Autodesk Inventor part; units mm, degrees
(part 4 of 13)
  line L1457 (42.6451, -0.0639) -> (42.8452, 0.1364) construction
  line L1458 (42.8452, 0.1364) -> (42.8452, 0.3832) construction
  spline S448 degree 3 poles (35.1829, 2.9373) (35.1829, 3.1841) (34.9826, 3.3841) (34.7358, 3.3841) knots 0 0 0 0 1 1 1 1
  line L1459 (35.1829, 2.9373) -> (35.1829, 3.1841) construction
  line L1460 (35.1829, 3.1841) -> (34.9826, 3.3841) construction
  line L1461 (34.9826, 3.3841) -> (34.7358, 3.3841) construction
  spline S449 degree 3 poles (34.7358, 3.3841) (34.4891, 3.3841) (34.289, 3.1841) (34.289, 2.9373) knots 0 0 0 0 1 1 1 1
  line L1462 (34.7358, 3.3841) -> (34.4891, 3.3841) construction
  line L1463 (34.4891, 3.3841) -> (34.289, 3.1841) construction
  line L1464 (34.289, 3.1841) -> (34.289, 2.9373) construction
  spline S450 degree 3 poles (34.289, 2.9373) (34.289, 2.6905) (34.4891, 2.4902) (34.7358, 2.4902) knots 0 0 0 0 1 1 1 1
  line L1465 (34.289, 2.9373) -> (34.289, 2.6905) construction
  line L1466 (34.289, 2.6905) -> (34.4891, 2.4902) construction
  line L1467 (34.4891, 2.4902) -> (34.7358, 2.4902) construction
  spline S451 degree 3 poles (34.7358, 2.4902) (34.9826, 2.4902) (35.1829, 2.6905) (35.1829, 2.9373) knots 0 0 0 0 1 1 1 1
  line L1468 (34.7358, 2.4902) -> (34.9826, 2.4902) construction
  line L1469 (34.9826, 2.4902) -> (35.1829, 2.6905) construction
  line L1470 (35.1829, 2.6905) -> (35.1829, 2.9373) construction
  spline S452 degree 3 poles (35.1829, 5.4914) (35.1829, 5.7382) (34.9826, 5.9382) (34.7358, 5.9382) knots 0 0 0 0 1 1 1 1
  line L1471 (35.1829, 5.4914) -> (35.1829, 5.7382) construction
  line L1472 (35.1829, 5.7382) -> (34.9826, 5.9382) construction
  line L1473 (34.9826, 5.9382) -> (34.7358, 5.9382) construction
  spline S453 degree 3 poles (34.7358, 5.9382) (34.4891, 5.9382) (34.289, 5.7382) (34.289, 5.4914) knots 0 0 0 0 1 1 1 1
  line L1474 (34.7358, 5.9382) -> (34.4891, 5.9382) construction
  line L1475 (34.4891, 5.9382) -> (34.289, 5.7382) construction
  line L1476 (34.289, 5.7382) -> (34.289, 5.4914) construction
  spline S454 degree 3 poles (34.289, 5.4914) (34.289, 5.2446) (34.4891, 5.0443) (34.7358, 5.0443) knots 0 0 0 0 1 1 1 1
  line L1477 (34.289, 5.4914) -> (34.289, 5.2446) construction
  line L1478 (34.289, 5.2446) -> (34.4891, 5.0443) construction
  line L1479 (34.4891, 5.0443) -> (34.7358, 5.0443) construction
  spline S455 degree 3 poles (34.7358, 5.0443) (34.9826, 5.0443) (35.1829, 5.2446) (35.1829, 5.4914) knots 0 0 0 0 1 1 1 1
  line L1480 (34.7358, 5.0443) -> (34.9826, 5.0443) construction
  line L1481 (34.9826, 5.0443) -> (35.1829, 5.2446) construction
  line L1482 (35.1829, 5.2446) -> (35.1829, 5.4914) construction
  spline S456 degree 3 poles (37.737, 5.4914) (37.737, 5.7382) (37.5369, 5.9382) (37.29, 5.9382) knots 0 0 0 0 1 1 1 1
  line L1483 (37.737, 5.4914) -> (37.737, 5.7382) construction
  line L1484 (37.737, 5.7382) -> (37.5369, 5.9382) construction
  line L1485 (37.5369, 5.9382) -> (37.29, 5.9382) construction
  spline S457 degree 3 poles (37.29, 5.9382) (37.0431, 5.9382) (36.843, 5.7382) (36.843, 5.4914) knots 0 0 0 0 1 1 1 1
  line L1486 (37.29, 5.9382) -> (37.0431, 5.9382) construction
  line L1487 (37.0431, 5.9382) -> (36.843, 5.7382) construction
  line L1488 (36.843, 5.7382) -> (36.843, 5.4914) construction
  spline S458 degree 3 poles (36.843, 5.4914) (36.843, 5.2446) (37.0431, 5.0443) (37.29, 5.0443) knots 0 0 0 0 1 1 1 1
  line L1489 (36.843, 5.4914) -> (36.843, 5.2446) construction
  line L1490 (36.843, 5.2446) -> (37.0431, 5.0443) construction
  line L1491 (37.0431, 5.0443) -> (37.29, 5.0443) construction
  spline S459 degree 3 poles (37.29, 5.0443) (37.5369, 5.0443) (37.737, 5.2446) (37.737, 5.4914) knots 0 0 0 0 1 1 1 1
  line L1492 (37.29, 5.0443) -> (37.5369, 5.0443) construction
  line L1493 (37.5369, 5.0443) -> (37.737, 5.2446) construction
  line L1494 (37.737, 5.2446) -> (37.737, 5.4914) construction
  spline S460 degree 3 poles (37.737, 0.3832) (37.737, 0.6299) (37.5369, 0.83) (37.29, 0.83) knots 0 0 0 0 1 1 1 1
  line L1495 (37.737, 0.3832) -> (37.737, 0.6299) construction
  line L1496 (37.737, 0.6299) -> (37.5369, 0.83) construction
  line L1497 (37.5369, 0.83) -> (37.29, 0.83) construction
  spline S461 degree 3 poles (37.29, 0.83) (37.0431, 0.83) (36.843, 0.6299) (36.843, 0.3832) knots 0 0 0 0 1 1 1 1
  line L1498 (37.29, 0.83) -> (37.0431, 0.83) construction
  line L1499 (37.0431, 0.83) -> (36.843, 0.6299) construction
  line L1500 (36.843, 0.6299) -> (36.843, 0.3832) construction
  spline S462 degree 3 poles (36.843, 0.3832) (36.843, 0.1364) (37.0431, -0.0639) (37.29, -0.0639) knots 0 0 0 0 1 1 1 1
  line L1501 (36.843, 0.3832) -> (36.843, 0.1364) construction
  line L1502 (36.843, 0.1364) -> (37.0431, -0.0639) construction
  line L1503 (37.0431, -0.0639) -> (37.29, -0.0639) construction
  spline S463 degree 3 poles (37.29, -0.0639) (37.5369, -0.0639) (37.737, 0.1364) (37.737, 0.3832) knots 0 0 0 0 1 1 1 1
  line L1504 (37.29, -0.0639) -> (37.5369, -0.0639) construction
  line L1505 (37.5369, -0.0639) -> (37.737, 0.1364) construction
  line L1506 (37.737, 0.1364) -> (37.737, 0.3832) construction
  spline S464 degree 3 poles (40.2911, 0.3832) (40.2911, 0.6299) (40.091, 0.83) (39.8441, 0.83) knots 0 0 0 0 1 1 1 1
  line L1507 (40.2911, 0.3832) -> (40.2911, 0.6299) construction
  line L1508 (40.2911, 0.6299) -> (40.091, 0.83) construction
  line L1509 (40.091, 0.83) -> (39.8441, 0.83) construction
  spline S465 degree 3 poles (39.8441, 0.83) (39.5972, 0.83) (39.3971, 0.6299) (39.3971, 0.3832) knots 0 0 0 0 1 1 1 1
  line L1510 (39.8441, 0.83) -> (39.5972, 0.83) construction
  line L1511 (39.5972, 0.83) -> (39.3971, 0.6299) construction
  line L1512 (39.3971, 0.6299) -> (39.3971, 0.3832) construction
  spline S466 degree 3 poles (39.3971, 0.3832) (39.3971, 0.1364) (39.5972, -0.0639) (39.8441, -0.0639) knots 0 0 0 0 1 1 1 1
  line L1513 (39.3971, 0.3832) -> (39.3971, 0.1364) construction
  line L1514 (39.3971, 0.1364) -> (39.5972, -0.0639) construction
  line L1515 (39.5972, -0.0639) -> (39.8441, -0.0639) construction
  spline S467 degree 3 poles (39.8441, -0.0639) (40.091, -0.0639) (40.2911, 0.1364) (40.2911, 0.3832) knots 0 0 0 0 1 1 1 1
  line L1516 (39.8441, -0.0639) -> (40.091, -0.0639) construction
  line L1517 (40.091, -0.0639) -> (40.2911, 0.1364) construction
  line L1518 (40.2911, 0.1364) -> (40.2911, 0.3832) construction
  spline S468 degree 3 poles (37.737, 2.9373) (37.737, 3.1841) (37.5369, 3.3841) (37.29, 3.3841) knots 0 0 0 0 1 1 1 1
  line L1519 (37.737, 2.9373) -> (37.737, 3.1841) construction
  line L1520 (37.737, 3.1841) -> (37.5369, 3.3841) construction
  line L1521 (37.5369, 3.3841) -> (37.29, 3.3841) construction
  spline S469 degree 3 poles (37.29, 3.3841) (37.0431, 3.3841) (36.843, 3.1841) (36.843, 2.9373) knots 0 0 0 0 1 1 1 1
  line L1522 (37.29, 3.3841) -> (37.0431, 3.3841) construction
  line L1523 (37.0431, 3.3841) -> (36.843, 3.1841) construction
  line L1524 (36.843, 3.1841) -> (36.843, 2.9373) construction
  spline S470 degree 3 poles (36.843, 2.9373) (36.843, 2.6905) (37.0431, 2.4902) (37.29, 2.4902) knots 0 0 0 0 1 1 1 1
  line L1525 (36.843, 2.9373) -> (36.843, 2.6905) construction
  line L1526 (36.843, 2.6905) -> (37.0431, 2.4902) construction
  line L1527 (37.0431, 2.4902) -> (37.29, 2.4902) construction
  spline S471 degree 3 poles (37.29, 2.4902) (37.5369, 2.4902) (37.737, 2.6905) (37.737, 2.9373) knots 0 0 0 0 1 1 1 1
  line L1528 (37.29, 2.4902) -> (37.5369, 2.4902) construction
  line L1529 (37.5369, 2.4902) -> (37.737, 2.6905) construction
  line L1530 (37.737, 2.6905) -> (37.737, 2.9373) construction
  spline S472 degree 3 poles (35.1829, 8.0455) (35.1829, 8.2923) (34.9826, 8.4923) (34.7358, 8.4923) knots 0 0 0 0 1 1 1 1
  line L1531 (35.1829, 8.0455) -> (35.1829, 8.2923) construction
  line L1532 (35.1829, 8.2923) -> (34.9826, 8.4923) construction
  line L1533 (34.9826, 8.4923) -> (34.7358, 8.4923) construction
  spline S473 degree 3 poles (34.7358, 8.4923) (34.4891, 8.4923) (34.289, 8.2923) (34.289, 8.0455) knots 0 0 0 0 1 1 1 1
  line L1534 (34.7358, 8.4923) -> (34.4891, 8.4923) construction
  line L1535 (34.4891, 8.4923) -> (34.289, 8.2923) construction
  line L1536 (34.289, 8.2923) -> (34.289, 8.0455) construction
  spline S474 degree 3 poles (34.289, 8.0455) (34.289, 7.7987) (34.4891, 7.5984) (34.7358, 7.5984) knots 0 0 0 0 1 1 1 1
  line L1537 (34.289, 8.0455) -> (34.289, 7.7987) construction
  line L1538 (34.289, 7.7987) -> (34.4891, 7.5984) construction
  line L1539 (34.4891, 7.5984) -> (34.7358, 7.5984) construction
  spline S475 degree 3 poles (34.7358, 7.5984) (34.9826, 7.5984) (35.1829, 7.7987) (35.1829, 8.0455) knots 0 0 0 0 1 1 1 1
  line L1540 (34.7358, 7.5984) -> (34.9826, 7.5984) construction
  line L1541 (34.9826, 7.5984) -> (35.1829, 7.7987) construction
  line L1542 (35.1829, 7.7987) -> (35.1829, 8.0455) construction
  spline S476 degree 3 poles (37.737, 8.0455) (37.737, 8.2923) (37.5369, 8.4923) (37.29, 8.4923) knots 0 0 0 0 1 1 1 1
  line L1543 (37.737, 8.0455) -> (37.737, 8.2923) construction
  line L1544 (37.737, 8.2923) -> (37.5369, 8.4923) construction
  line L1545 (37.5369, 8.4923) -> (37.29, 8.4923) construction
  spline S477 degree 3 poles (37.29, 8.4923) (37.0431, 8.4923) (36.843, 8.2923) (36.843, 8.0455) knots 0 0 0 0 1 1 1 1
  line L1546 (37.29, 8.4923) -> (37.0431, 8.4923) construction
  line L1547 (37.0431, 8.4923) -> (36.843, 8.2923) construction
  line L1548 (36.843, 8.2923) -> (36.843, 8.0455) construction
  spline S478 degree 3 poles (36.843, 8.0455) (36.843, 7.7987) (37.0431, 7.5984) (37.29, 7.5984) knots 0 0 0 0 1 1 1 1
  line L1549 (36.843, 8.0455) -> (36.843, 7.7987) construction
  line L1550 (36.843, 7.7987) -> (37.0431, 7.5984) construction
  line L1551 (37.0431, 7.5984) -> (37.29, 7.5984) construction
  spline S479 degree 3 poles (37.29, 7.5984) (37.5369, 7.5984) (37.737, 7.7987) (37.737, 8.0455) knots 0 0 0 0 1 1 1 1
  line L1552 (37.29, 7.5984) -> (37.5369, 7.5984) construction
  line L1553 (37.5369, 7.5984) -> (37.737, 7.7987) construction
  line L1554 (37.737, 7.7987) -> (37.737, 8.0455) construction
  spline S480 degree 3 poles (35.1829, 10.5996) (35.1829, 10.8464) (34.9826, 11.0465) (34.7358, 11.0465) knots 0 0 0 0 1 1 1 1
  line L1555 (35.1829, 10.5996) -> (35.1829, 10.8464) construction
  line L1556 (35.1829, 10.8464) -> (34.9826, 11.0465) construction
  line L1557 (34.9826, 11.0465) -> (34.7358, 11.0465) construction
  spline S481 degree 3 poles (34.7358, 11.0465) (34.4891, 11.0465) (34.289, 10.8464) (34.289, 10.5996) knots 0 0 0 0 1 1 1 1
  line L1558 (34.7358, 11.0465) -> (34.4891, 11.0465) construction
  line L1559 (34.4891, 11.0465) -> (34.289, 10.8464) construction
  line L1560 (34.289, 10.8464) -> (34.289, 10.5996) construction
  spline S482 degree 3 poles (34.289, 10.5996) (34.289, 10.3528) (34.4891, 10.1525) (34.7358, 10.1525) knots 0 0 0 0 1 1 1 1
  line L1561 (34.289, 10.5996) -> (34.289, 10.3528) construction
  line L1562 (34.289, 10.3528) -> (34.4891, 10.1525) construction
  line L1563 (34.4891, 10.1525) -> (34.7358, 10.1525) construction
  spline S483 degree 3 poles (34.7358, 10.1525) (34.9826, 10.1525) (35.1829, 10.3528) (35.1829, 10.5996) knots 0 0 0 0 1 1 1 1
  line L1564 (34.7358, 10.1525) -> (34.9826, 10.1525) construction
  line L1565 (34.9826, 10.1525) -> (35.1829, 10.3528) construction
  line L1566 (35.1829, 10.3528) -> (35.1829, 10.5996) construction
  spline S484 degree 3 poles (37.737, 10.5996) (37.737, 10.8464) (37.5369, 11.0465) (37.29, 11.0465) knots 0 0 0 0 1 1 1 1
  line L1567 (37.737, 10.5996) -> (37.737, 10.8464) construction
  line L1568 (37.737, 10.8464) -> (37.5369, 11.0465) construction
  line L1569 (37.5369, 11.0465) -> (37.29, 11.0465) construction
  spline S485 degree 3 poles (37.29, 11.0465) (37.0431, 11.0465) (36.843, 10.8464) (36.843, 10.5996) knots 0 0 0 0 1 1 1 1
  line L1570 (37.29, 11.0465) -> (37.0431, 11.0465) construction
  line L1571 (37.0431, 11.0465) -> (36.843, 10.8464) construction
  line L1572 (36.843, 10.8464) -> (36.843, 10.5996) construction
  spline S486 degree 3 poles (36.843, 10.5996) (36.843, 10.3528) (37.0431, 10.1525) (37.29, 10.1525) knots 0 0 0 0 1 1 1 1
  line L1573 (36.843, 10.5996) -> (36.843, 10.3528) construction
  line L1574 (36.843, 10.3528) -> (37.0431, 10.1525) construction
  line L1575 (37.0431, 10.1525) -> (37.29, 10.1525) construction
  spline S487 degree 3 poles (37.29, 10.1525) (37.5369, 10.1525) (37.737, 10.3528) (37.737, 10.5996) knots 0 0 0 0 1 1 1 1
  line L1576 (37.29, 10.1525) -> (37.5369, 10.1525) construction
  line L1577 (37.5369, 10.1525) -> (37.737, 10.3528) construction
  line L1578 (37.737, 10.3528) -> (37.737, 10.5996) construction
  spline S488 degree 3 poles (35.1829, 13.1537) (35.1829, 13.4005) (34.9826, 13.6006) (34.7358, 13.6006) knots 0 0 0 0 1 1 1 1
  line L1579 (35.1829, 13.1537) -> (35.1829, 13.4005) construction
  line L1580 (35.1829, 13.4005) -> (34.9826, 13.6006) construction
  line L1581 (34.9826, 13.6006) -> (34.7358, 13.6006) construction
  spline S489 degree 3 poles (34.7358, 13.6006) (34.4891, 13.6006) (34.289, 13.4005) (34.289, 13.1537) knots 0 0 0 0 1 1 1 1
  line L1582 (34.7358, 13.6006) -> (34.4891, 13.6006) construction
  line L1583 (34.4891, 13.6006) -> (34.289, 13.4005) construction
  line L1584 (34.289, 13.4005) -> (34.289, 13.1537) construction
  spline S490 degree 3 poles (34.289, 13.1537) (34.289, 12.9069) (34.4891, 12.7067) (34.7358, 12.7067) knots 0 0 0 0 1 1 1 1
  line L1585 (34.289, 13.1537) -> (34.289, 12.9069) construction
  line L1586 (34.289, 12.9069) -> (34.4891, 12.7067) construction
  line L1587 (34.4891, 12.7067) -> (34.7358, 12.7067) construction
  spline S491 degree 3 poles (34.7358, 12.7067) (34.9826, 12.7067) (35.1829, 12.9069) (35.1829, 13.1537) knots 0 0 0 0 1 1 1 1
  line L1588 (34.7358, 12.7067) -> (34.9826, 12.7067) construction
  line L1589 (34.9826, 12.7067) -> (35.1829, 12.9069) construction
  line L1590 (35.1829, 12.9069) -> (35.1829, 13.1537) construction
  spline S492 degree 3 poles (37.737, 13.1537) (37.737, 13.4005) (37.5369, 13.6006) (37.29, 13.6006) knots 0 0 0 0 1 1 1 1
  line L1591 (37.737, 13.1537) -> (37.737, 13.4005) construction
  line L1592 (37.737, 13.4005) -> (37.5369, 13.6006) construction
  line L1593 (37.5369, 13.6006) -> (37.29, 13.6006) construction
  spline S493 degree 3 poles (37.29, 13.6006) (37.0431, 13.6006) (36.843, 13.4005) (36.843, 13.1537) knots 0 0 0 0 1 1 1 1
  line L1594 (37.29, 13.6006) -> (37.0431, 13.6006) construction
  line L1595 (37.0431, 13.6006) -> (36.843, 13.4005) construction
  line L1596 (36.843, 13.4005) -> (36.843, 13.1537) construction
  spline S494 degree 3 poles (36.843, 13.1537) (36.843, 12.9069) (37.0431, 12.7067) (37.29, 12.7067) knots 0 0 0 0 1 1 1 1
  line L1597 (36.843, 13.1537) -> (36.843, 12.9069) construction
  line L1598 (36.843, 12.9069) -> (37.0431, 12.7067) construction
  line L1599 (37.0431, 12.7067) -> (37.29, 12.7067) construction
  spline S495 degree 3 poles (37.29, 12.7067) (37.5369, 12.7067) (37.737, 12.9069) (37.737, 13.1537) knots 0 0 0 0 1 1 1 1
  line L1600 (37.29, 12.7067) -> (37.5369, 12.7067) construction
  line L1601 (37.5369, 12.7067) -> (37.737, 12.9069) construction
  line L1602 (37.737, 12.9069) -> (37.737, 13.1537) construction
  spline S496 degree 3 poles (35.1829, 15.7078) (35.1829, 15.9546) (34.9826, 16.1547) (34.7358, 16.1547) knots 0 0 0 0 1 1 1 1
  line L1603 (35.1829, 15.7078) -> (35.1829, 15.9546) construction
  line L1604 (35.1829, 15.9546) -> (34.9826, 16.1547) construction
  line L1605 (34.9826, 16.1547) -> (34.7358, 16.1547) construction
  spline S497 degree 3 poles (34.7358, 16.1547) (34.4891, 16.1547) (34.289, 15.9546) (34.289, 15.7078) knots 0 0 0 0 1 1 1 1
  line L1606 (34.7358, 16.1547) -> (34.4891, 16.1547) construction
  line L1607 (34.4891, 16.1547) -> (34.289, 15.9546) construction
  line L1608 (34.289, 15.9546) -> (34.289, 15.7078) construction
  spline S498 degree 3 poles (34.289, 15.7078) (34.289, 15.461) (34.4891, 15.2608) (34.7358, 15.2608) knots 0 0 0 0 1 1 1 1
  line L1609 (34.289, 15.7078) -> (34.289, 15.461) construction
  line L1610 (34.289, 15.461) -> (34.4891, 15.2608) construction
  line L1611 (34.4891, 15.2608) -> (34.7358, 15.2608) construction
  spline S499 degree 3 poles (34.7358, 15.2608) (34.9826, 15.2608) (35.1829, 15.461) (35.1829, 15.7078) knots 0 0 0 0 1 1 1 1
  line L1612 (34.7358, 15.2608) -> (34.9826, 15.2608) construction
  line L1613 (34.9826, 15.2608) -> (35.1829, 15.461) construction
  line L1614 (35.1829, 15.461) -> (35.1829, 15.7078) construction
  spline S500 degree 3 poles (37.737, 15.7078) (37.737, 15.9546) (37.5369, 16.1547) (37.29, 16.1547) knots 0 0 0 0 1 1 1 1
  line L1615 (37.737, 15.7078) -> (37.737, 15.9546) construction
  line L1616 (37.737, 15.9546) -> (37.5369, 16.1547) construction
  line L1617 (37.5369, 16.1547) -> (37.29, 16.1547) construction
  spline S501 degree 3 poles (37.29, 16.1547) (37.0431, 16.1547) (36.843, 15.9546) (36.843, 15.7078) knots 0 0 0 0 1 1 1 1
  line L1618 (37.29, 16.1547) -> (37.0431, 16.1547) construction
  line L1619 (37.0431, 16.1547) -> (36.843, 15.9546) construction
  line L1620 (36.843, 15.9546) -> (36.843, 15.7078) construction
  spline S502 degree 3 poles (36.843, 15.7078) (36.843, 15.461) (37.0431, 15.2608) (37.29, 15.2608) knots 0 0 0 0 1 1 1 1
  line L1621 (36.843, 15.7078) -> (36.843, 15.461) construction
  line L1622 (36.843, 15.461) -> (37.0431, 15.2608) construction
  line L1623 (37.0431, 15.2608) -> (37.29, 15.2608) construction
  spline S503 degree 3 poles (37.29, 15.2608) (37.5369, 15.2608) (37.737, 15.461) (37.737, 15.7078) knots 0 0 0 0 1 1 1 1
  line L1624 (37.29, 15.2608) -> (37.5369, 15.2608) construction
  line L1625 (37.5369, 15.2608) -> (37.737, 15.461) construction
  line L1626 (37.737, 15.461) -> (37.737, 15.7078) construction
  spline S504 degree 3 poles (35.1829, 18.2619) (35.1829, 18.5087) (34.9826, 18.7088) (34.7358, 18.7088) knots 0 0 0 0 1 1 1 1
  line L1627 (35.1829, 18.2619) -> (35.1829, 18.5087) construction
  line L1628 (35.1829, 18.5087) -> (34.9826, 18.7088) construction
  line L1629 (34.9826, 18.7088) -> (34.7358, 18.7088) construction
  spline S505 degree 3 poles (34.7358, 18.7088) (34.4891, 18.7088) (34.289, 18.5087) (34.289, 18.2619) knots 0 0 0 0 1 1 1 1
  line L1630 (34.7358, 18.7088) -> (34.4891, 18.7088) construction
  line L1631 (34.4891, 18.7088) -> (34.289, 18.5087) construction
  line L1632 (34.289, 18.5087) -> (34.289, 18.2619) construction
  spline S506 degree 3 poles (34.289, 18.2619) (34.289, 18.0151) (34.4891, 17.8149) (34.7358, 17.8149) knots 0 0 0 0 1 1 1 1
  line L1633 (34.289, 18.2619) -> (34.289, 18.0151) construction
  line L1634 (34.289, 18.0151) -> (34.4891, 17.8149) construction
  line L1635 (34.4891, 17.8149) -> (34.7358, 17.8149) construction
  spline S507 degree 3 poles (34.7358, 17.8149) (34.9826, 17.8149) (35.1829, 18.0151) (35.1829, 18.2619) knots 0 0 0 0 1 1 1 1
  line L1636 (34.7358, 17.8149) -> (34.9826, 17.8149) construction
  line L1637 (34.9826, 17.8149) -> (35.1829, 18.0151) construction
  line L1638 (35.1829, 18.0151) -> (35.1829, 18.2619) construction
  spline S508 degree 3 poles (37.737, 18.2619) (37.737, 18.5087) (37.5369, 18.7088) (37.29, 18.7088) knots 0 0 0 0 1 1 1 1
  line L1639 (37.737, 18.2619) -> (37.737, 18.5087) construction
  line L1640 (37.737, 18.5087) -> (37.5369, 18.7088) construction
  line L1641 (37.5369, 18.7088) -> (37.29, 18.7088) construction
  spline S509 degree 3 poles (37.29, 18.7088) (37.0431, 18.7088) (36.843, 18.5087) (36.843, 18.2619) knots 0 0 0 0 1 1 1 1
  line L1642 (37.29, 18.7088) -> (37.0431, 18.7088) construction
  line L1643 (37.0431, 18.7088) -> (36.843, 18.5087) construction
  line L1644 (36.843, 18.5087) -> (36.843, 18.2619) construction
  spline S510 degree 3 poles (36.843, 18.2619) (36.843, 18.0151) (37.0431, 17.8149) (37.29, 17.8149) knots 0 0 0 0 1 1 1 1
  line L1645 (36.843, 18.2619) -> (36.843, 18.0151) construction
  line L1646 (36.843, 18.0151) -> (37.0431, 17.8149) construction
  line L1647 (37.0431, 17.8149) -> (37.29, 17.8149) construction
  spline S511 degree 3 poles (37.29, 17.8149) (37.5369, 17.8149) (37.737, 18.0151) (37.737, 18.2619) knots 0 0 0 0 1 1 1 1
  line L1648 (37.29, 17.8149) -> (37.5369, 17.8149) construction
  line L1649 (37.5369, 17.8149) -> (37.737, 18.0151) construction
  line L1650 (37.737, 18.0151) -> (37.737, 18.2619) construction
  spline S512 degree 3 poles (35.1829, 20.816) (35.1829, 21.0628) (34.9826, 21.2629) (34.7358, 21.2629) knots 0 0 0 0 1 1 1 1
  line L1651 (35.1829, 20.816) -> (35.1829, 21.0628) construction
  line L1652 (35.1829, 21.0628) -> (34.9826, 21.2629) construction
  line L1653 (34.9826, 21.2629) -> (34.7358, 21.2629) construction
  spline S513 degree 3 poles (34.7358, 21.2629) (34.4891, 21.2629) (34.289, 21.0628) (34.289, 20.816) knots 0 0 0 0 1 1 1 1
  line L1654 (34.7358, 21.2629) -> (34.4891, 21.2629) construction
  line L1655 (34.4891, 21.2629) -> (34.289, 21.0628) construction
  line L1656 (34.289, 21.0628) -> (34.289, 20.816) construction
  spline S514 degree 3 poles (34.289, 20.816) (34.289, 20.5692) (34.4891, 20.369) (34.7358, 20.369) knots 0 0 0 0 1 1 1 1
  line L1657 (34.289, 20.816) -> (34.289, 20.5692) construction
  line L1658 (34.289, 20.5692) -> (34.4891, 20.369) construction
  line L1659 (34.4891, 20.369) -> (34.7358, 20.369) construction
  spline S515 degree 3 poles (34.7358, 20.369) (34.9826, 20.369) (35.1829, 20.5692) (35.1829, 20.816) knots 0 0 0 0 1 1 1 1
  line L1660 (34.7358, 20.369) -> (34.9826, 20.369) construction
  line L1661 (34.9826, 20.369) -> (35.1829, 20.5692) construction
  line L1662 (35.1829, 20.5692) -> (35.1829, 20.816) construction
  spline S516 degree 3 poles (35.1829, 23.3701) (35.1829, 23.6169) (34.9826, 23.817) (34.7358, 23.817) knots 0 0 0 0 1 1 1 1
  line L1663 (35.1829, 23.3701) -> (35.1829, 23.6169) construction
  line L1664 (35.1829, 23.6169) -> (34.9826, 23.817) construction
  line L1665 (34.9826, 23.817) -> (34.7358, 23.817) construction
  spline S517 degree 3 poles (34.7358, 23.817) (34.4891, 23.817) (34.289, 23.6169) (34.289, 23.3701) knots 0 0 0 0 1 1 1 1
  line L1666 (34.7358, 23.817) -> (34.4891, 23.817) construction
  line L1667 (34.4891, 23.817) -> (34.289, 23.6169) construction
  line L1668 (34.289, 23.6169) -> (34.289, 23.3701) construction
  spline S518 degree 3 poles (34.289, 23.3701) (34.289, 23.1233) (34.4891, 22.9231) (34.7358, 22.9231) knots 0 0 0 0 1 1 1 1
  line L1669 (34.289, 23.3701) -> (34.289, 23.1233) construction
  line L1670 (34.289, 23.1233) -> (34.4891, 22.9231) construction
  line L1671 (34.4891, 22.9231) -> (34.7358, 22.9231) construction
  spline S519 degree 3 poles (34.7358, 22.9231) (34.9826, 22.9231) (35.1829, 23.1233) (35.1829, 23.3701) knots 0 0 0 0 1 1 1 1
  line L1672 (34.7358, 22.9231) -> (34.9826, 22.9231) construction
  line L1673 (34.9826, 22.9231) -> (35.1829, 23.1233) construction
  line L1674 (35.1829, 23.1233) -> (35.1829, 23.3701) construction
  spline S520 degree 3 poles (35.1829, 25.9242) (35.1829, 26.171) (34.9826, 26.3711) (34.7358, 26.3711) knots 0 0 0 0 1 1 1 1
  line L1675 (35.1829, 25.9242) -> (35.1829, 26.171) construction
  line L1676 (35.1829, 26.171) -> (34.9826, 26.3711) construction
  line L1677 (34.9826, 26.3711) -> (34.7358, 26.3711) construction
  spline S521 degree 3 poles (34.7358, 26.3711) (34.4891, 26.3711) (34.289, 26.171) (34.289, 25.9242) knots 0 0 0 0 1 1 1 1
  line L1678 (34.7358, 26.3711) -> (34.4891, 26.3711) construction
  line L1679 (34.4891, 26.3711) -> (34.289, 26.171) construction
  line L1680 (34.289, 26.171) -> (34.289, 25.9242) construction
  spline S522 degree 3 poles (34.289, 25.9242) (34.289, 25.6775) (34.4891, 25.4772) (34.7358, 25.4772) knots 0 0 0 0 1 1 1 1
  line L1681 (34.289, 25.9242) -> (34.289, 25.6775) construction
  line L1682 (34.289, 25.6775) -> (34.4891, 25.4772) construction
  line L1683 (34.4891, 25.4772) -> (34.7358, 25.4772) construction
  spline S523 degree 3 poles (34.7358, 25.4772) (34.9826, 25.4772) (35.1829, 25.6775) (35.1829, 25.9242) knots 0 0 0 0 1 1 1 1
  line L1684 (34.7358, 25.4772) -> (34.9826, 25.4772) construction
  line L1685 (34.9826, 25.4772) -> (35.1829, 25.6775) construction
  line L1686 (35.1829, 25.6775) -> (35.1829, 25.9242) construction
  spline S524 degree 3 poles (35.1829, 28.4784) (35.1829, 28.7251) (34.9826, 28.9252) (34.7358, 28.9252) knots 0 0 0 0 1 1 1 1
  line L1687 (35.1829, 28.4784) -> (35.1829, 28.7251) construction
  line L1688 (35.1829, 28.7251) -> (34.9826, 28.9252) construction
  line L1689 (34.9826, 28.9252) -> (34.7358, 28.9252) construction
  spline S525 degree 3 poles (34.7358, 28.9252) (34.4891, 28.9252) (34.289, 28.7251) (34.289, 28.4784) knots 0 0 0 0 1 1 1 1
  line L1690 (34.7358, 28.9252) -> (34.4891, 28.9252) construction
  line L1691 (34.4891, 28.9252) -> (34.289, 28.7251) construction
  line L1692 (34.289, 28.7251) -> (34.289, 28.4784) construction
  spline S526 degree 3 poles (34.289, 28.4784) (34.289, 28.2316) (34.4891, 28.0313) (34.7358, 28.0313) knots 0 0 0 0 1 1 1 1
  line L1693 (34.289, 28.4784) -> (34.289, 28.2316) construction
  line L1694 (34.289, 28.2316) -> (34.4891, 28.0313) construction
  line L1695 (34.4891, 28.0313) -> (34.7358, 28.0313) construction
  spline S527 degree 3 poles (34.7358, 28.0313) (34.9826, 28.0313) (35.1829, 28.2316) (35.1829, 28.4784) knots 0 0 0 0 1 1 1 1
  line L1696 (34.7358, 28.0313) -> (34.9826, 28.0313) construction
  line L1697 (34.9826, 28.0313) -> (35.1829, 28.2316) construction
  line L1698 (35.1829, 28.2316) -> (35.1829, 28.4784) construction
  spline S528 degree 3 poles (35.1829, 31.0325) (35.1829, 31.2793) (34.9826, 31.4793) (34.7358, 31.4793) knots 0 0 0 0 1 1 1 1
  line L1699 (35.1829, 31.0325) -> (35.1829, 31.2793) construction
  line L1700 (35.1829, 31.2793) -> (34.9826, 31.4793) construction
  line L1701 (34.9826, 31.4793) -> (34.7358, 31.4793) construction
  spline S529 degree 3 poles (34.7358, 31.4793) (34.4891, 31.4793) (34.289, 31.2793) (34.289, 31.0325) knots 0 0 0 0 1 1 1 1
  line L1702 (34.7358, 31.4793) -> (34.4891, 31.4793) construction
  line L1703 (34.4891, 31.4793) -> (34.289, 31.2793) construction
  line L1704 (34.289, 31.2793) -> (34.289, 31.0325) construction
  spline S530 degree 3 poles (34.289, 31.0325) (34.289, 30.7857) (34.4891, 30.5854) (34.7358, 30.5854) knots 0 0 0 0 1 1 1 1
  line L1705 (34.289, 31.0325) -> (34.289, 30.7857) construction
  line L1706 (34.289, 30.7857) -> (34.4891, 30.5854) construction
  line L1707 (34.4891, 30.5854) -> (34.7358, 30.5854) construction
  spline S531 degree 3 poles (34.7358, 30.5854) (34.9826, 30.5854) (35.1829, 30.7857) (35.1829, 31.0325) knots 0 0 0 0 1 1 1 1
  line L1708 (34.7358, 30.5854) -> (34.9826, 30.5854) construction
  line L1709 (34.9826, 30.5854) -> (35.1829, 30.7857) construction
  line L1710 (35.1829, 30.7857) -> (35.1829, 31.0325) construction
  spline S532 degree 3 poles (37.737, 20.816) (37.737, 21.0628) (37.5369, 21.2629) (37.29, 21.2629) knots 0 0 0 0 1 1 1 1
  line L1711 (37.737, 20.816) -> (37.737, 21.0628) construction
  line L1712 (37.737, 21.0628) -> (37.5369, 21.2629) construction
  line L1713 (37.5369, 21.2629) -> (37.29, 21.2629) construction
  spline S533 degree 3 poles (37.29, 21.2629) (37.0431, 21.2629) (36.843, 21.0628) (36.843, 20.816) knots 0 0 0 0 1 1 1 1
  line L1714 (37.29, 21.2629) -> (37.0431, 21.2629) construction
  line L1715 (37.0431, 21.2629) -> (36.843, 21.0628) construction
  line L1716 (36.843, 21.0628) -> (36.843, 20.816) construction
  spline S534 degree 3 poles (36.843, 20.816) (36.843, 20.5692) (37.0431, 20.369) (37.29, 20.369) knots 0 0 0 0 1 1 1 1
  line L1717 (36.843, 20.816) -> (36.843, 20.5692) construction
  line L1718 (36.843, 20.5692) -> (37.0431, 20.369) construction
  line L1719 (37.0431, 20.369) -> (37.29, 20.369) construction
  spline S535 degree 3 poles (37.29, 20.369) (37.5369, 20.369) (37.737, 20.5692) (37.737, 20.816) knots 0 0 0 0 1 1 1 1
  line L1720 (37.29, 20.369) -> (37.5369, 20.369) construction
  line L1721 (37.5369, 20.369) -> (37.737, 20.5692) construction
  line L1722 (37.737, 20.5692) -> (37.737, 20.816) construction
  spline S536 degree 3 poles (37.737, 23.3701) (37.737, 23.6169) (37.5369, 23.817) (37.29, 23.817) knots 0 0 0 0 1 1 1 1
  line L1723 (37.737, 23.3701) -> (37.737, 23.6169) construction
  line L1724 (37.737, 23.6169) -> (37.5369, 23.817) construction
  line L1725 (37.5369, 23.817) -> (37.29, 23.817) construction
  spline S537 degree 3 poles (37.29, 23.817) (37.0431, 23.817) (36.843, 23.6169) (36.843, 23.3701) knots 0 0 0 0 1 1 1 1
  line L1726 (37.29, 23.817) -> (37.0431, 23.817) construction
  line L1727 (37.0431, 23.817) -> (36.843, 23.6169) construction
  line L1728 (36.843, 23.6169) -> (36.843, 23.3701) construction
  spline S538 degree 3 poles (36.843, 23.3701) (36.843, 23.1233) (37.0431, 22.9231) (37.29, 22.9231) knots 0 0 0 0 1 1 1 1
  line L1729 (36.843, 23.3701) -> (36.843, 23.1233) construction
  line L1730 (36.843, 23.1233) -> (37.0431, 22.9231) construction
  line L1731 (37.0431, 22.9231) -> (37.29, 22.9231) construction
  spline S539 degree 3 poles (37.29, 22.9231) (37.5369, 22.9231) (37.737, 23.1233) (37.737, 23.3701) knots 0 0 0 0 1 1 1 1
  line L1732 (37.29, 22.9231) -> (37.5369, 22.9231) construction
  line L1733 (37.5369, 22.9231) -> (37.737, 23.1233) construction
  line L1734 (37.737, 23.1233) -> (37.737, 23.3701) construction
  spline S540 degree 3 poles (37.737, 25.9242) (37.737, 26.171) (37.5369, 26.3711) (37.29, 26.3711) knots 0 0 0 0 1 1 1 1
  line L1735 (37.737, 25.9242) -> (37.737, 26.171) construction
  line L1736 (37.737, 26.171) -> (37.5369, 26.3711) construction
  line L1737 (37.5369, 26.3711) -> (37.29, 26.3711) construction
  spline S541 degree 3 poles (37.29, 26.3711) (37.0431, 26.3711) (36.843, 26.171) (36.843, 25.9242) knots 0 0 0 0 1 1 1 1
  line L1738 (37.29, 26.3711) -> (37.0431, 26.3711) construction
  line L1739 (37.0431, 26.3711) -> (36.843, 26.171) construction
  line L1740 (36.843, 26.171) -> (36.843, 25.9242) construction
  spline S542 degree 3 poles (36.843, 25.9242) (36.843, 25.6775) (37.0431, 25.4772) (37.29, 25.4772) knots 0 0 0 0 1 1 1 1
  line L1741 (36.843, 25.9242) -> (36.843, 25.6775) construction
  line L1742 (36.843, 25.6775) -> (37.0431, 25.4772) construction
  line L1743 (37.0431, 25.4772) -> (37.29, 25.4772) construction
  spline S543 degree 3 poles (37.29, 25.4772) (37.5369, 25.4772) (37.737, 25.6775) (37.737, 25.9242) knots 0 0 0 0 1 1 1 1
  line L1744 (37.29, 25.4772) -> (37.5369, 25.4772) construction
  line L1745 (37.5369, 25.4772) -> (37.737, 25.6775) construction
  line L1746 (37.737, 25.6775) -> (37.737, 25.9242) construction
  spline S544 degree 3 poles (37.737, 28.4784) (37.737, 28.7251) (37.5369, 28.9252) (37.29, 28.9252) knots 0 0 0 0 1 1 1 1
  line L1747 (37.737, 28.4784) -> (37.737, 28.7251) construction
  line L1748 (37.737, 28.7251) -> (37.5369, 28.9252) construction
  line L1749 (37.5369, 28.9252) -> (37.29, 28.9252) construction
  spline S545 degree 3 poles (37.29, 28.9252) (37.0431, 28.9252) (36.843, 28.7251) (36.843, 28.4784) knots 0 0 0 0 1 1 1 1
  line L1750 (37.29, 28.9252) -> (37.0431, 28.9252) construction
  line L1751 (37.0431, 28.9252) -> (36.843, 28.7251) construction
  line L1752 (36.843, 28.7251) -> (36.843, 28.4784) construction
  spline S546 degree 3 poles (36.843, 28.4784) (36.843, 28.2316) (37.0431, 28.0313) (37.29, 28.0313) knots 0 0 0 0 1 1 1 1
  line L1753 (36.843, 28.4784) -> (36.843, 28.2316) construction
  line L1754 (36.843, 28.2316) -> (37.0431, 28.0313) construction
  line L1755 (37.0431, 28.0313) -> (37.29, 28.0313) construction
  spline S547 degree 3 poles (37.29, 28.0313) (37.5369, 28.0313) (37.737, 28.2316) (37.737, 28.4784) knots 0 0 0 0 1 1 1 1
  line L1756 (37.29, 28.0313) -> (37.5369, 28.0313) construction
  line L1757 (37.5369, 28.0313) -> (37.737, 28.2316) construction
  line L1758 (37.737, 28.2316) -> (37.737, 28.4784) construction
  spline S548 degree 3 poles (37.737, 31.0325) (37.737, 31.2793) (37.5369, 31.4793) (37.29, 31.4793) knots 0 0 0 0 1 1 1 1
  line L1759 (37.737, 31.0325) -> (37.737, 31.2793) construction
  line L1760 (37.737, 31.2793) -> (37.5369, 31.4793) construction
  line L1761 (37.5369, 31.4793) -> (37.29, 31.4793) construction
  spline S549 degree 3 poles (37.29, 31.4793) (37.0431, 31.4793) (36.843, 31.2793) (36.843, 31.0325) knots 0 0 0 0 1 1 1 1
  line L1762 (37.29, 31.4793) -> (37.0431, 31.4793) construction
  line L1763 (37.0431, 31.4793) -> (36.843, 31.2793) construction
  line L1764 (36.843, 31.2793) -> (36.843, 31.0325) construction
  spline S550 degree 3 poles (36.843, 31.0325) (36.843, 30.7857) (37.0431, 30.5854) (37.29, 30.5854) knots 0 0 0 0 1 1 1 1
  line L1765 (36.843, 31.0325) -> (36.843, 30.7857) construction
  line L1766 (36.843, 30.7857) -> (37.0431, 30.5854) construction
  line L1767 (37.0431, 30.5854) -> (37.29, 30.5854) construction
  spline S551 degree 3 poles (37.29, 30.5854) (37.5369, 30.5854) (37.737, 30.7857) (37.737, 31.0325) knots 0 0 0 0 1 1 1 1
  line L1768 (37.29, 30.5854) -> (37.5369, 30.5854) construction
  line L1769 (37.5369, 30.5854) -> (37.737, 30.7857) construction
  line L1770 (37.737, 30.7857) -> (37.737, 31.0325) construction
  spline S552 degree 3 poles (45.3993, 0.3832) (45.3993, 0.6299) (45.1992, 0.83) (44.9523, 0.83) knots 0 0 0 0 1 1 1 1
  line L1771 (45.3993, 0.3832) -> (45.3993, 0.6299) construction
  line L1772 (45.3993, 0.6299) -> (45.1992, 0.83) construction
  line L1773 (45.1992, 0.83) -> (44.9523, 0.83) construction
  spline S553 degree 3 poles (44.9523, 0.83) (44.7054, 0.83) (44.5054, 0.6299) (44.5054, 0.3832) knots 0 0 0 0 1 1 1 1
  line L1774 (44.9523, 0.83) -> (44.7054, 0.83) construction
  line L1775 (44.7054, 0.83) -> (44.5054, 0.6299) construction
  line L1776 (44.5054, 0.6299) -> (44.5054, 0.3832) construction
  spline S554 degree 3 poles (44.5054, 0.3832) (44.5054, 0.1364) (44.7054, -0.0639) (44.9523, -0.0639) knots 0 0 0 0 1 1 1 1
  line L1777 (44.5054, 0.3832) -> (44.5054, 0.1364) construction
  line L1778 (44.5054, 0.1364) -> (44.7054, -0.0639) construction
  line L1779 (44.7054, -0.0639) -> (44.9523, -0.0639) construction
  spline S555 degree 3 poles (44.9523, -0.0639) (45.1992, -0.0639) (45.3993, 0.1364) (45.3993, 0.3832) knots 0 0 0 0 1 1 1 1
  line L1780 (44.9523, -0.0639) -> (45.1992, -0.0639) construction
  line L1781 (45.1992, -0.0639) -> (45.3993, 0.1364) construction
  line L1782 (45.3993, 0.1364) -> (45.3993, 0.3832) construction
  spline S556 degree 3 poles (47.9534, 0.3832) (47.9534, 0.6299) (47.7533, 0.83) (47.5064, 0.83) knots 0 0 0 0 1 1 1 1
  line L1783 (47.9534, 0.3832) -> (47.9534, 0.6299) construction
  line L1784 (47.9534, 0.6299) -> (47.7533, 0.83) construction
  line L1785 (47.7533, 0.83) -> (47.5064, 0.83) construction
  spline S557 degree 3 poles (47.5064, 0.83) (47.2595, 0.83) (47.0595, 0.6299) (47.0595, 0.3832) knots 0 0 0 0 1 1 1 1
  line L1786 (47.5064, 0.83) -> (47.2595, 0.83) construction
  line L1787 (47.2595, 0.83) -> (47.0595, 0.6299) construction
  line L1788 (47.0595, 0.6299) -> (47.0595, 0.3832) construction
  spline S558 degree 3 poles (47.0595, 0.3832) (47.0595, 0.1364) (47.2595, -0.0639) (47.5064, -0.0639) knots 0 0 0 0 1 1 1 1
  line L1789 (47.0595, 0.3832) -> (47.0595, 0.1364) construction
  line L1790 (47.0595, 0.1364) -> (47.2595, -0.0639) construction
  line L1791 (47.2595, -0.0639) -> (47.5064, -0.0639) construction
  spline S559 degree 3 poles (47.5064, -0.0639) (47.7533, -0.0639) (47.9534, 0.1364) (47.9534, 0.3832) knots 0 0 0 0 1 1 1 1
  line L1792 (47.5064, -0.0639) -> (47.7533, -0.0639) construction
  line L1793 (47.7533, -0.0639) -> (47.9534, 0.1364) construction
  line L1794 (47.9534, 0.1364) -> (47.9534, 0.3832) construction
  spline S560 degree 3 poles (46.6763, 9.7057) (46.6763, 10.5872) (45.9615, 11.302) (45.08, 11.302) knots 0 0 0 0 1 1 1 1
  line L1795 (46.6763, 9.7057) -> (46.6763, 10.5872) construction
  line L1796 (46.6763, 10.5872) -> (45.9615, 11.302) construction
  line L1797 (45.9615, 11.302) -> (45.08, 11.302) construction
  spline S561 degree 3 poles (45.08, 11.302) (44.1985, 11.302) (43.4837, 10.5872) (43.4837, 9.7057) knots 0 0 0 0 1 1 1 1
  line L1798 (45.08, 11.302) -> (44.1985, 11.302) construction
  line L1799 (44.1985, 11.302) -> (43.4837, 10.5872) construction
  line L1800 (43.4837, 10.5872) -> (43.4837, 9.7057) construction
  spline S562 degree 3 poles (43.4837, 9.7057) (43.4837, 8.8241) (44.1985, 8.1094) (45.08, 8.1094) knots 0 0 0 0 1 1 1 1
  line L1801 (43.4837, 9.7057) -> (43.4837, 8.8241) construction
  line L1802 (43.4837, 8.8241) -> (44.1985, 8.1094) construction
  line L1803 (44.1985, 8.1094) -> (45.08, 8.1094) construction
  spline S563 degree 3 poles (45.08, 8.1094) (45.9615, 8.1094) (46.6763, 8.8241) (46.6763, 9.7057) knots 0 0 0 0 1 1 1 1
  line L1804 (45.08, 8.1094) -> (45.9615, 8.1094) construction
  line L1805 (45.9615, 8.1094) -> (46.6763, 8.8241) construction
  line L1806 (46.6763, 8.8241) -> (46.6763, 9.7057) construction
  spline S564 degree 3 poles (52.8701, 9.7057) (52.8701, 10.4814) (52.2411, 11.1103) (51.4653, 11.1103) knots 0 0 0 0 1 1 1 1
  line L1807 (52.8701, 9.7057) -> (52.8701, 10.4814) construction
  line L1808 (52.8701, 10.4814) -> (52.2411, 11.1103) construction
  line L1809 (52.2411, 11.1103) -> (51.4653, 11.1103) construction
  spline S565 degree 3 poles (51.4653, 11.1103) (50.6895, 11.1103) (50.0605, 10.4814) (50.0605, 9.7057) knots 0 0 0 0 1 1 1 1
  line L1810 (51.4653, 11.1103) -> (50.6895, 11.1103) construction
  line L1811 (50.6895, 11.1103) -> (50.0605, 10.4814) construction
  line L1812 (50.0605, 10.4814) -> (50.0605, 9.7057) construction
  spline S566 degree 3 poles (50.0605, 9.7057) (50.0605, 8.9299) (50.6895, 8.3009) (51.4653, 8.3009) knots 0 0 0 0 1 1 1 1
  line L1813 (50.0605, 9.7057) -> (50.0605, 8.9299) construction
  line L1814 (50.0605, 8.9299) -> (50.6895, 8.3009) construction
  line L1815 (50.6895, 8.3009) -> (51.4653, 8.3009) construction
  spline S567 degree 3 poles (51.4653, 8.3009) (52.2411, 8.3009) (52.8701, 8.9299) (52.8701, 9.7057) knots 0 0 0 0 1 1 1 1
  line L1816 (51.4653, 8.3009) -> (52.2411, 8.3009) construction
  line L1817 (52.2411, 8.3009) -> (52.8701, 8.9299) construction
  line L1818 (52.8701, 8.9299) -> (52.8701, 9.7057) construction
  spline S568 degree 3 poles (49.6774, 14.303) (49.6774, 15.0787) (49.0485, 15.7078) (48.2727, 15.7078) knots 0 0 0 0 1 1 1 1
  line L1819 (49.6774, 14.303) -> (49.6774, 15.0787) construction
  line L1820 (49.6774, 15.0787) -> (49.0485, 15.7078) construction
  line L1821 (49.0485, 15.7078) -> (48.2727, 15.7078) construction
  spline S569 degree 3 poles (48.2727, 15.7078) (47.4969, 15.7078) (46.8679, 15.0787) (46.8679, 14.303) knots 0 0 0 0 1 1 1 1
  line L1822 (48.2727, 15.7078) -> (47.4969, 15.7078) construction
  line L1823 (47.4969, 15.7078) -> (46.8679, 15.0787) construction
  line L1824 (46.8679, 15.0787) -> (46.8679, 14.303) construction
  spline S570 degree 3 poles (46.8679, 14.303) (46.8679, 13.5273) (47.4969, 12.8983) (48.2727, 12.8983) knots 0 0 0 0 1 1 1 1
  line L1825 (46.8679, 14.303) -> (46.8679, 13.5273) construction
  line L1826 (46.8679, 13.5273) -> (47.4969, 12.8983) construction
  line L1827 (47.4969, 12.8983) -> (48.2727, 12.8983) construction
  spline S571 degree 3 poles (48.2727, 12.8983) (49.0485, 12.8983) (49.6774, 13.5273) (49.6774, 14.303) knots 0 0 0 0 1 1 1 1
  line L1828 (48.2727, 12.8983) -> (49.0485, 12.8983) construction
  line L1829 (49.0485, 12.8983) -> (49.6774, 13.5273) construction
  line L1830 (49.6774, 13.5273) -> (49.6774, 14.303) construction
  spline S572 degree 3 poles (9.6418, 0.3832) (9.6418, 0.6299) (9.4415, 0.83) (9.1948, 0.83) knots 0 0 0 0 1 1 1 1
  line L1831 (9.6418, 0.3832) -> (9.6418, 0.6299) construction
  line L1832 (9.6418, 0.6299) -> (9.4415, 0.83) construction
  line L1833 (9.4415, 0.83) -> (9.1948, 0.83) construction
  spline S573 degree 3 poles (9.1948, 0.83) (8.948, 0.83) (8.7479, 0.6299) (8.7479, 0.3832) knots 0 0 0 0 1 1 1 1
  line L1834 (9.1948, 0.83) -> (8.948, 0.83) construction
  line L1835 (8.948, 0.83) -> (8.7479, 0.6299) construction
  line L1836 (8.7479, 0.6299) -> (8.7479, 0.3832) construction
  spline S574 degree 3 poles (8.7479, 0.3832) (8.7479, 0.1364) (8.948, -0.0639) (9.1948, -0.0639) knots 0 0 0 0 1 1 1 1
  line L1837 (8.7479, 0.3832) -> (8.7479, 0.1364) construction
  line L1838 (8.7479, 0.1364) -> (8.948, -0.0639) construction
  line L1839 (8.948, -0.0639) -> (9.1948, -0.0639) construction
  spline S575 degree 3 poles (9.1948, -0.0639) (9.4415, -0.0639) (9.6418, 0.1364) (9.6418, 0.3832) knots 0 0 0 0 1 1 1 1
  line L1840 (9.1948, -0.0639) -> (9.4415, -0.0639) construction
  line L1841 (9.4415, -0.0639) -> (9.6418, 0.1364) construction
  line L1842 (9.6418, 0.1364) -> (9.6418, 0.3832) construction
  spline S576 degree 3 poles (12.1959, 0.3832) (12.1959, 0.6299) (11.9957, 0.83) (11.7489, 0.83) knots 0 0 0 0 1 1 1 1
  line L1843 (12.1959, 0.3832) -> (12.1959, 0.6299) construction
  line L1844 (12.1959, 0.6299) -> (11.9957, 0.83) construction
  line L1845 (11.9957, 0.83) -> (11.7489, 0.83) construction
  spline S577 degree 3 poles (11.7489, 0.83) (11.5021, 0.83) (11.302, 0.6299) (11.302, 0.3832) knots 0 0 0 0 1 1 1 1
  line L1846 (11.7489, 0.83) -> (11.5021, 0.83) construction
  line L1847 (11.5021, 0.83) -> (11.302, 0.6299) construction
  line L1848 (11.302, 0.6299) -> (11.302, 0.3832) construction
  spline S578 degree 3 poles (11.302, 0.3832) (11.302, 0.1364) (11.5021, -0.0639) (11.7489, -0.0639) knots 0 0 0 0 1 1 1 1
  line L1849 (11.302, 0.3832) -> (11.302, 0.1364) construction
  line L1850 (11.302, 0.1364) -> (11.5021, -0.0639) construction
  line L1851 (11.5021, -0.0639) -> (11.7489, -0.0639) construction
  spline S579 degree 3 poles (11.7489, -0.0639) (11.9957, -0.0639) (12.1959, 0.1364) (12.1959, 0.3832) knots 0 0 0 0 1 1 1 1
  line L1852 (11.7489, -0.0639) -> (11.9957, -0.0639) construction
  line L1853 (11.9957, -0.0639) -> (12.1959, 0.1364) construction
  line L1854 (12.1959, 0.1364) -> (12.1959, 0.3832) construction
  spline S580 degree 3 poles (14.75, 0.3832) (14.75, 0.6299) (14.5498, 0.83) (14.303, 0.83) knots 0 0 0 0 1 1 1 1
  line L1855 (14.75, 0.3832) -> (14.75, 0.6299) construction
  line L1856 (14.75, 0.6299) -> (14.5498, 0.83) construction
  line L1857 (14.5498, 0.83) -> (14.303, 0.83) construction
  spline S581 degree 3 poles (14.303, 0.83) (14.0562, 0.83) (13.8561, 0.6299) (13.8561, 0.3832) knots 0 0 0 0 1 1 1 1
  line L1858 (14.303, 0.83) -> (14.0562, 0.83) construction
  line L1859 (14.0562, 0.83) -> (13.8561, 0.6299) construction
  line L1860 (13.8561, 0.6299) -> (13.8561, 0.3832) construction
  spline S582 degree 3 poles (13.8561, 0.3832) (13.8561, 0.1364) (14.0562, -0.0639) (14.303, -0.0639) knots 0 0 0 0 1 1 1 1
  line L1861 (13.8561, 0.3832) -> (13.8561, 0.1364) construction
  line L1862 (13.8561, 0.1364) -> (14.0562, -0.0639) construction
  line L1863 (14.0562, -0.0639) -> (14.303, -0.0639) construction
  spline S583 degree 3 poles (14.303, -0.0639) (14.5498, -0.0639) (14.75, 0.1364) (14.75, 0.3832) knots 0 0 0 0 1 1 1 1
  line L1864 (14.303, -0.0639) -> (14.5498, -0.0639) construction
  line L1865 (14.5498, -0.0639) -> (14.75, 0.1364) construction
  line L1866 (14.75, 0.1364) -> (14.75, 0.3832) construction
  spline S584 degree 3 poles (17.3041, 0.3832) (17.3041, 0.6299) (17.1039, 0.83) (16.8571, 0.83) knots 0 0 0 0 1 1 1 1
  line L1867 (17.3041, 0.3832) -> (17.3041, 0.6299) construction
  line L1868 (17.3041, 0.6299) -> (17.1039, 0.83) construction
  line L1869 (17.1039, 0.83) -> (16.8571, 0.83) construction
  spline S585 degree 3 poles (16.8571, 0.83) (16.6103, 0.83) (16.4102, 0.6299) (16.4102, 0.3832) knots 0 0 0 0 1 1 1 1
  line L1870 (16.8571, 0.83) -> (16.6103, 0.83) construction
  line L1871 (16.6103, 0.83) -> (16.4102, 0.6299) construction
  line L1872 (16.4102, 0.6299) -> (16.4102, 0.3832) construction
  spline S586 degree 3 poles (16.4102, 0.3832) (16.4102, 0.1364) (16.6103, -0.0639) (16.8571, -0.0639) knots 0 0 0 0 1 1 1 1
  line L1873 (16.4102, 0.3832) -> (16.4102, 0.1364) construction
  line L1874 (16.4102, 0.1364) -> (16.6103, -0.0639) construction
  line L1875 (16.6103, -0.0639) -> (16.8571, -0.0639) construction
  spline S587 degree 3 poles (16.8571, -0.0639) (17.1039, -0.0639) (17.3041, 0.1364) (17.3041, 0.3832) knots 0 0 0 0 1 1 1 1
  line L1876 (16.8571, -0.0639) -> (17.1039, -0.0639) construction
  line L1877 (17.1039, -0.0639) -> (17.3041, 0.1364) construction
  line L1878 (17.3041, 0.1364) -> (17.3041, 0.3832) construction
  spline S588 degree 3 poles (17.3041, 2.9373) (17.3041, 3.1841) (17.1039, 3.3841) (16.8571, 3.3841) knots 0 0 0 0 1 1 1 1
  line L1879 (17.3041, 2.9373) -> (17.3041, 3.1841) construction
  line L1880 (17.3041, 3.1841) -> (17.1039, 3.3841) construction
  line L1881 (17.1039, 3.3841) -> (16.8571, 3.3841) construction
  spline S589 degree 3 poles (16.8571, 3.3841) (16.6103, 3.3841) (16.4102, 3.1841) (16.4102, 2.9373) knots 0 0 0 0 1 1 1 1
  line L1882 (16.8571, 3.3841) -> (16.6103, 3.3841) construction
  line L1883 (16.6103, 3.3841) -> (16.4102, 3.1841) construction
  line L1884 (16.4102, 3.1841) -> (16.4102, 2.9373) construction
  spline S590 degree 3 poles (16.4102, 2.9373) (16.4102, 2.6905) (16.6103, 2.4902) (16.8571, 2.4902) knots 0 0 0 0 1 1 1 1
  line L1885 (16.4102, 2.9373) -> (16.4102, 2.6905) construction
  line L1886 (16.4102, 2.6905) -> (16.6103, 2.4902) construction
  line L1887 (16.6103, 2.4902) -> (16.8571, 2.4902) construction
  spline S591 degree 3 poles (16.8571, 2.4902) (17.1039, 2.4902) (17.3041, 2.6905) (17.3041, 2.9373) knots 0 0 0 0 1 1 1 1
  line L1888 (16.8571, 2.4902) -> (17.1039, 2.4902) construction
  line L1889 (17.1039, 2.4902) -> (17.3041, 2.6905) construction
  line L1890 (17.3041, 2.6905) -> (17.3041, 2.9373) construction
  spline S592 degree 3 poles (19.8582, 2.9373) (19.8582, 3.1841) (19.658, 3.3841) (19.4112, 3.3841) knots 0 0 0 0 1 1 1 1
  line L1891 (19.8582, 2.9373) -> (19.8582, 3.1841) construction
  line L1892 (19.8582, 3.1841) -> (19.658, 3.3841) construction
  line L1893 (19.658, 3.3841) -> (19.4112, 3.3841) construction
  spline S593 degree 3 poles (19.4112, 3.3841) (19.1644, 3.3841) (18.9643, 3.1841) (18.9643, 2.9373) knots 0 0 0 0 1 1 1 1
  line L1894 (19.4112, 3.3841) -> (19.1644, 3.3841) construction
  line L1895 (19.1644, 3.3841) -> (18.9643, 3.1841) construction
  line L1896 (18.9643, 3.1841) -> (18.9643, 2.9373) construction
  spline S594 degree 3 poles (18.9643, 2.9373) (18.9643, 2.6905) (19.1644, 2.4902) (19.4112, 2.4902) knots 0 0 0 0 1 1 1 1
  line L1897 (18.9643, 2.9373) -> (18.9643, 2.6905) construction
  line L1898 (18.9643, 2.6905) -> (19.1644, 2.4902) construction
  line L1899 (19.1644, 2.4902) -> (19.4112, 2.4902) construction
  spline S595 degree 3 poles (19.4112, 2.4902) (19.658, 2.4902) (19.8582, 2.6905) (19.8582, 2.9373) knots 0 0 0 0 1 1 1 1
  line L1900 (19.4112, 2.4902) -> (19.658, 2.4902) construction
  line L1901 (19.658, 2.4902) -> (19.8582, 2.6905) construction
  line L1902 (19.8582, 2.6905) -> (19.8582, 2.9373) construction
  spline S596 degree 3 poles (26.2435, 0.3832) (26.2435, 0.6299) (26.0433, 0.83) (25.7965, 0.83) knots 0 0 0 0 1 1 1 1
  line L1903 (26.2435, 0.3832) -> (26.2435, 0.6299) construction
  line L1904 (26.2435, 0.6299) -> (26.0433, 0.83) construction
  line L1905 (26.0433, 0.83) -> (25.7965, 0.83) construction
  spline S597 degree 3 poles (25.7965, 0.83) (25.5497, 0.83) (25.3496, 0.6299) (25.3496, 0.3832) knots 0 0 0 0 1 1 1 1
  line L1906 (25.7965, 0.83) -> (25.5497, 0.83) construction
  line L1907 (25.5497, 0.83) -> (25.3496, 0.6299) construction
  line L1908 (25.3496, 0.6299) -> (25.3496, 0.3832) construction
  spline S598 degree 3 poles (25.3496, 0.3832) (25.3496, 0.1364) (25.5497, -0.0639) (25.7965, -0.0639) knots 0 0 0 0 1 1 1 1
  line L1909 (25.3496, 0.3832) -> (25.3496, 0.1364) construction
  line L1910 (25.3496, 0.1364) -> (25.5497, -0.0639) construction
  line L1911 (25.5497, -0.0639) -> (25.7965, -0.0639) construction
  spline S599 degree 3 poles (25.7965, -0.0639) (26.0433, -0.0639) (26.2435, 0.1364) (26.2435, 0.3832) knots 0 0 0 0 1 1 1 1
  line L1912 (25.7965, -0.0639) -> (26.0433, -0.0639) construction
  line L1913 (26.0433, -0.0639) -> (26.2435, 0.1364) construction
  line L1914 (26.2435, 0.1364) -> (26.2435, 0.3832) construction
  spline S600 degree 3 poles (23.6894, 0.3832) (23.6894, 0.6299) (23.4891, 0.83) (23.2424, 0.83) knots 0 0 0 0 1 1 1 1
  line L1915 (23.6894, 0.3832) -> (23.6894, 0.6299) construction
  line L1916 (23.6894, 0.6299) -> (23.4891, 0.83) construction
  line L1917 (23.4891, 0.83) -> (23.2424, 0.83) construction
  spline S601 degree 3 poles (23.2424, 0.83) (22.9956, 0.83) (22.7955, 0.6299) (22.7955, 0.3832) knots 0 0 0 0 1 1 1 1
  line L1918 (23.2424, 0.83) -> (22.9956, 0.83) construction
  line L1919 (22.9956, 0.83) -> (22.7955, 0.6299) construction
  line L1920 (22.7955, 0.6299) -> (22.7955, 0.3832) construction
  spline S602 degree 3 poles (22.7955, 0.3832) (22.7955, 0.1364) (22.9956, -0.0639) (23.2424, -0.0639) knots 0 0 0 0 1 1 1 1
  line L1921 (22.7955, 0.3832) -> (22.7955, 0.1364) construction
  line L1922 (22.7955, 0.1364) -> (22.9956, -0.0639) construction
  line L1923 (22.9956, -0.0639) -> (23.2424, -0.0639) construction
  spline S603 degree 3 poles (23.2424, -0.0639) (23.4891, -0.0639) (23.6894, 0.1364) (23.6894, 0.3832) knots 0 0 0 0 1 1 1 1
  line L1924 (23.2424, -0.0639) -> (23.4891, -0.0639) construction
  line L1925 (23.4891, -0.0639) -> (23.6894, 0.1364) construction
  line L1926 (23.6894, 0.1364) -> (23.6894, 0.3832) construction
  spline S604 degree 3 poles (21.1353, 0.3832) (21.1353, 0.6299) (20.935, 0.83) (20.6882, 0.83) knots 0 0 0 0 1 1 1 1
  line L1927 (21.1353, 0.3832) -> (21.1353, 0.6299) construction
  line L1928 (21.1353, 0.6299) -> (20.935, 0.83) construction